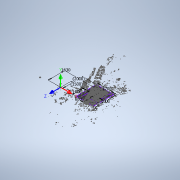
# Autodesk Inventor part: leonOSM
Saved by Autodesk Inventor 2021 (Build 250183000, 183)
## iProperties
Created: 2021-06-19
Part Number: leonOSM
Material: Genérico
Document SubType Name: Modeling
Designer: luise
Density: 1 g/cm^3
Appearance: Valor por defecto
Author: luise
Autodesk Inventor part; units mm, degrees
ref_plane "YZ Plane" through (0, 0, 0) normal (1, 0, 0) x (0, 1, 0)
ref_plane "XZ Plane" through (0, 0, 0) normal (0, 1, 0) x (-1, 0, 0)
ref_plane "XY Plane" through (0, 0, 0) normal (0, 0, 1) x (1, 0, 0)
sketch "Boceto1" plane through (0, 0, 0) normal (0, 1, 0) x (-1, 0, 0)
  line L0 (-1500000, -2000000) -> (-3200000, -2000000)
  line L1 (-3200000, -2000000) -> (-3200000, 0)
  line L2 (-3200000, 0) -> (-1500000, 0)
  line L3 (-1500000, 0) -> (-1500000, -2000000)
  point P0 (0, 0)
  dimension "d7" = 1700000
  dimension "d9" = 2000000
  constraints: 8 end point, 2 parallel, 1 horizontal, 1 perpendicular
  measures "d7" distance between parallel lines of L1 L3
  measures "d9" distance between parallel lines of L2 L0
extrude "Extrusión1" add sketch "Boceto1" against normal blind 1000
sketch "Boceto3" plane through (0, 0, 0) normal (0, 1, 0) x (1, 0, 0)
  line L0 (1500000, 0) -> (3200000, 0) projected
  line L1 (3200000, 0) -> (3200000, 2000000) projected
  line L2 (3200000, 2000000) -> (1500000, 2000000) projected
  line L3 (1500000, 2000000) -> (1500000, 0) projected
  line L4 (3200000, 0) -> (1500000, 0) projected
  line L5 (1500000, 0) -> (1500000, 2000000) projected
  line L6 (3200000, 2000000) -> (3200000, 0) projected
  line L7 (1500000, 2000000) -> (2350000, 2000000)
  line L8 (1500000, 1000000) -> (1500000, 2000000)
  line L9 (3200000, 1000000) -> (3200000, 2000000)
  line L10 (3200000, 2000000) -> (2350000, 2000000)
  line L11 (1500000, 1000000) -> (1500000, 0)
  line L12 (1500000, 0) -> (2350000, 0)
  line L13 (3200000, 1000000) -> (3200000, 0)
  line L14 (3200000, 0) -> (2350000, 0)
  line L15 (1500000, 2000000) -> (3200000, 2000000) projected
  line L16 (1500000, 1000000) -> (3200000, 1000000)
  line L17 (1500000, 1630000) -> (2350000, 1630000)
  line L18 (2350000, 1000000) -> (1500000, 1000000)
  line L19 (1500000, 1000000) -> (1500000, 1630000)
  line L20 (2350000, 2000000) -> (2954055, 2000000)
  line L21 (2954055, 2000000) -> (2954055, 1000000)
  line L22 (2954055, 1000000) -> (2350000, 1000000)
  line L23 (1809479, 1000000) -> (2350000, 1000000)
  line L24 (2350000, 1000000) -> (2350000, 0)
  line L25 (2350000, 0) -> (1809479, 0)
  line L26 (1809479, 0) -> (1809479, 1000000)
  line L27 (3200000, 459725) -> (2350000, 459725)
  line L28 (2350000, 459725) -> (2350000, 1000000)
  line L29 (2350000, 1000000) -> (3200000, 1000000)
  line L30 (3200000, 1000000) -> (3200000, 459725)
  line L31 (2350000, 1000000) -> (2350000, 2000000)
  point P0 (0, 0)
  dimension "d14" = 1500000
  dimension "d15" = 2000000
  dimension "d17" = 1630000
  dimension "d18" = 1000000
  dimension "d19" = 850000
  constraints: 48 end point, 6 parallel, 5 horizontal, 4 perpendicular, 4 point on line, 1 midpoint, 1 vertical
  measures "d14" distance from line of point (0, 0) L3
  measures "d15" distance from line of point (0, 0) L7
  measures "d17" distance from line of point (0, 0) L17
  measures "d18" distance between parallel lines of L0 L16
  measures "d19" distance between parallel lines of L24 L3
